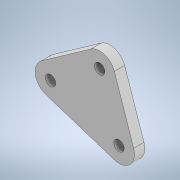
# Autodesk Inventor part: 後ろウィング固定フレーム押さえ
Saved by Autodesk Inventor 2020.2 (Build 242310000, 310)
## iProperties
Created: 2020-05-06
Part Number: 後ろウィング固定フレーム押さえ
Material: 一般
Document SubType Name: Modeling
Designer: mozar
Density: 1 g/cm^3
Appearance: 既定
Author: mozar
Autodesk Inventor part; units mm, degrees
ref_plane "YZ Plane" through (0, 0, 0) normal (1, 0, 0) x (0, 1, 0)
ref_plane "XZ Plane" through (0, 0, 0) normal (0, 1, 0) x (-1, 0, 0)
ref_plane "XY Plane" through (0, 0, 0) normal (0, 0, 1) x (1, 0, 0)
sketch "スケッチ1" plane through (0, 0, 0) normal (0, 0, 1) x (1, 0, 0)
  circle A0 centre (117.5177, -35.5687) radius 1.5
  circle A1 centre (95.4507, -12.9865) radius 1.5
  circle A2 centre (97.5945, -29.101) radius 1.5
  circle A3 centre (111.885, -19) radius 1.5
  line L0 (116.6369, -13.86) -> (104.8897, -3)
  line L1 (104.8897, -3) -> (101.885, -3)
  arc A4 (99.885, -3) -> (101.885, -3) centre (100.885, -3) ccw
  line L2 (99.885, -3) -> (99.885, 0)
  line L3 (99.885, 0) -> (84.885, 0)
  line L4 (84.885, 0) -> (84.885, -3)
  arc A5 (82.885, -3) -> (84.885, -3) centre (83.885, -3) ccw
  line L5 (82.885, -3) -> (81.4397, -3)
  arc A6 (79.4397, -3) -> (81.4397, -3) centre (80.4397, -3) ccw
  line L6 (79.4397, -3) -> (79.4397, 0)
  line L7 (79.4397, 0) -> (64.4397, 0)
  line L8 (64.4397, 0) -> (64.4397, -3)
  arc A7 (62.4397, -3) -> (64.4397, -3) centre (63.4397, -3) ccw
  line L9 (62.4397, -3) -> (59.4397, -3)
  line L10 (59.4397, -3) -> (59.4397, -6)
  line L11 (59.4397, -6) -> (65.1115, -8.2188)
  arc A8 (65.1115, -8.2188) -> (69.3788, -9.8882) centre (68.4397, -6) ccw
  line L12 (69.3788, -9.8882) -> (97.5091, -20.8927)
  arc A9 (97.5091, -20.8927) -> (98.5543, -24.7045) centre (111.885, -19) ccw
  arc A10 (98.5543, -24.7045) -> (97.6262, -33.6009) centre (97.5945, -29.101) ccw
  line L13 (97.6262, -33.6009) -> (107.1669, -33.5336)
  line L14 (107.1669, -33.5336) -> (114.849, -39.192)
  arc A11 (114.849, -39.192) -> (121.9415, -34.7438) centre (117.5177, -35.5687) ccw
  line L15 (121.9415, -34.7438) -> (118.7664, -17.7168)
  arc A12 (118.7664, -17.7168) -> (116.6369, -13.86) centre (111.885, -19) ccw
  line L16 (69.4397, -3) -> (74.4397, -3)
  arc A13 (76.4397, -3) -> (74.4397, -3) centre (75.4397, -3) ccw
  line L17 (76.4397, -3) -> (76.4397, -6)
  arc A14 (74.4397, -6) -> (76.4397, -6) centre (75.4397, -6) ccw
  line L18 (74.4397, -6) -> (69.4397, -6)
  arc A15 (67.4397, -6) -> (69.4397, -6) centre (68.4397, -6) ccw
  line L19 (67.4397, -6) -> (67.4397, -3)
  arc A16 (69.4397, -3) -> (67.4397, -3) centre (68.4397, -3) ccw
  arc A17 (94.885, -6) -> (96.885, -6) centre (95.885, -6) ccw
  line L20 (94.885, -6) -> (89.885, -6)
  arc A18 (87.885, -6) -> (89.885, -6) centre (88.885, -6) ccw
  line L21 (87.885, -6) -> (87.885, -3)
  arc A19 (89.885, -3) -> (87.885, -3) centre (88.885, -3) ccw
  line L22 (89.885, -3) -> (94.885, -3)
  arc A20 (96.885, -3) -> (94.885, -3) centre (95.885, -3) ccw
  line L23 (96.885, -3) -> (96.885, -6)
  circle A21 centre (97.5945, -29.101) radius 4.5
  circle A22 centre (111.885, -19) radius 4.5
  circle A23 centre (117.5177, -35.5687) radius 4.5
  line L24 (94.9971, -25.4263) -> (109.2877, -15.3253)
  line L25 (116.1456, -17.5516) -> (121.7783, -34.1203)
  line L26 (116.1283, -39.8488) -> (96.205, -33.3811)
  point P0 (0, 0)
  point P1 (0, 0)
  dimension "d0" = 9
  constraints: 54 end point, 42 point on circle, 24 centre point, 9 horizontal, 9 vertical, 6 tangent, 3 coincident, 91 other
  measures "d0" diameter of A22
extrude "押し出し1" add sketch "スケッチ1" against normal blind 3 contours A11 A23 | A23 L14 L13 A21 A9 L24 A22 L25 | L26 A10 L13 L14 A11 | A22 | A10 A21 | L24 A9 A10
sketch "スケッチ2" plane through (0, 0, -3) normal (0, 0, -1) x (-1, 0, 0)
  line L0 (-94.9971, -25.4263) -> (-109.2877, -15.3253) projected
  arc A0 (-109.2877, -15.3253) -> (-116.1456, -17.5516) centre (-111.885, -19) ccw projected
  line L1 (-116.1456, -17.5516) -> (-121.7783, -34.1203) projected
  arc A1 (-121.7783, -34.1203) -> (-116.1283, -39.8488) centre (-117.5177, -35.5687) ccw projected
  line L2 (-116.1283, -39.8488) -> (-96.205, -33.3811) projected
  arc A2 (-96.205, -33.3811) -> (-94.9971, -25.4263) centre (-97.5945, -29.101) ccw projected
  circle A3 centre (-111.885, -19) radius 1.5 projected
  circle A4 centre (-97.5945, -29.101) radius 1.5 projected
  circle A5 centre (-117.5177, -35.5687) radius 1.5 projected
  circle A6 centre (-97.5945, -29.101) radius 1.5 projected
  circle A7 centre (-97.5945, -29.101) radius 3
  circle A8 centre (-111.885, -19) radius 1.5 projected
  circle A9 centre (-111.885, -19) radius 3
  circle A10 centre (-117.5177, -35.5687) radius 1.5 projected
  circle A11 centre (-117.5177, -35.5687) radius 3
  point P0 (0, 0)
  dimension "d3" = 6
  dimension "d4" = 6
  dimension "d6" = 6
  constraints: 3 centre point, 3 coincident
  measures "d3" diameter of A7
  measures "d4" diameter of A9
  measures "d6" diameter of A11
extrude "押し出し2" cut sketch "スケッチ2" against normal blind 0.4 contours A5 | A7 | A9 | A11
